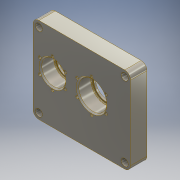
# Autodesk Inventor part: корпус01
Saved by Autodesk Inventor 2016 (Build 200138000, 138)
## iProperties
Created: 2021-04-22
Part Number: корпус01
Material: Типовые
Document SubType Name: Modeling
Designer: Лол
Density: 1 g/cm^3
Appearance: Титан — полированный
Author: Лол
Autodesk Inventor part; units mm, degrees
ref_plane "YZ Plane" through (0, 0, 0) normal (1, 0, 0) x (0, 1, 0)
ref_plane "XZ Plane" through (0, 0, 0) normal (0, 1, 0) x (-1, 0, 0)
ref_plane "XY Plane" through (0, 0, 0) normal (0, 0, 1) x (1, 0, 0)
sketch "Эскиз1" plane through (0, 0, 0) normal (0, 0, 1) x (1, 0, 0)
  line L0 (0, -65.4) -> (0, 10.9) projected
  line L1 (-170, 0) -> (180, 0) projected
  line L2 (-120, -12.5) -> (-120, -54.5)
  line L3 (-120, -54.5) -> (130, -54.5)
  line L4 (130, -54.5) -> (130, -12.5)
  line L5 (130, -12.5) -> (-120, -12.5)
  point P0 (0, 0)
  dimension "d0" = 12.5
  dimension "d1" = 250
  dimension "d2" = 42
  dimension "d3" = 120
  constraints: 8 end point, 3 perpendicular, 1 vertical
  measures "d0" distance between parallel lines of L5 L1
  measures "d1" distance of L2.end L3.end
  measures "d2" distance of L2.start L2.end
  measures "d3" distance between parallel lines of L2 L0
extrude "Выдавливание1" add sketch "Эскиз1" along normal blind 100 and the other way blind 120
sketch "Эскиз3" plane through (-120, -54.5, 100) normal (0, -1, 0) x (1, 0, 0)
  line L0 (120, -264) -> (120, 44) projected
  line L1 (-50, -100) -> (300, -100) projected
  circle A0 centre (150, -100) radius 36
  circle A1 centre (50, -100) radius 31
  point P0 (120, -100)
  dimension "d6" = 72
  dimension "d7" = 62
  dimension "d8" = 100
  dimension "d9" = 70
  constraints: 2 centre point, 2 point on line
  measures "d6" diameter of A0
  measures "d7" diameter of A1
  measures "d8" distance of A0.centre A1.centre
  measures "d9" distance from line of L0 A1.centre
extrude "Выдавливание2" cut sketch "Эскиз3" against normal blind 37
sketch "Эскиз4" plane through (-120, -54.5, 100) normal (0, -1, 0) x (1, 0, 0)
  line L0 (120, -264) -> (120, 44) projected
  line L1 (-50, -100) -> (300, -100) projected
  circle A0 centre (50, -100) radius 31 projected
  circle A1 centre (150, -100) radius 36 projected
  circle A2 centre (50, -100) radius 27
  circle A3 centre (150, -100) radius 31.5
  point P0 (120, -100)
  dimension "d12" = 63
  dimension "d13" = 54
  constraints: 2 centre point, 2 coincident
  measures "d12" diameter of A3
  measures "d13" diameter of A2
extrude "Выдавливание3" cut sketch "Эскиз4" against normal through all contours A3 L1 L0 | L0 L1 A3 | L1 A3 L0 | L0 A3 L1 | A2 L1 | L1 A2
sketch "Эскиз5" plane through (-120, -12.5, 100) normal (0, 1, 0) x (1, 0, 0)
  line L0 (120, 264) -> (120, -44) projected
  line L1 (-50, 100) -> (300, 100) projected
  circle A0 centre (150, 100) radius 31.5 projected
  circle A1 centre (50, 100) radius 27 projected
  arc A2 (86.0774, 126.8964) -> (86.0774, 73.1036) centre (50, 100) ccw
  arc A3 (108.2641, 72.4661) -> (108.2641, 127.5339) centre (150, 100) ccw
  arc A4 (86.0774, 126.8964) -> (108.2641, 127.5339) centre (96.9471, 135) ccw
  arc A5 (108.2641, 72.4661) -> (86.0774, 73.1036) centre (96.9471, 65) ccw
  line L2 (250, 220) -> (250, 0) projected
  line L3 (0, 220) -> (250, 220) projected
  line L4 (0, 0) -> (0, 220) projected
  line L5 (250, 0) -> (0, 0) projected
  line L6 (26, 214) -> (224, 214)
  line L7 (244, 194) -> (244, 26)
  line L8 (224, 6) -> (26, 6)
  line L9 (6, 26) -> (6, 194)
  arc A6 (244, 194) -> (224, 214) centre (224, 194) ccw
  arc A7 (26, 214) -> (6, 194) centre (26, 194) ccw
  arc A8 (6, 26) -> (26, 6) centre (26, 26) ccw
  arc A9 (224, 6) -> (244, 26) centre (224, 26) ccw
  point P0 (120, 100)
  dimension "d16" = 100
  dimension "d17" = 90
  dimension "d18" = 35
  dimension "d19" = 35
  dimension "d20" = 6
  dimension "d21" = 6
  dimension "d22" = 6
  dimension "d23" = 6
  dimension "d24" = 20
  constraints: 16 point on circle, 12 tangent, 8 centre point, 8 end point, 3 equal radius, 2 coincident, 2 parallel, 1 horizontal, 1 perpendicular
  measures "d16" diameter of A3
  measures "d17" diameter of A2
  measures "d18" distance from line of A4.centre L1
  measures "d19" distance from line of A5.centre L1
  measures "d20" distance between parallel lines of L7 L2
  measures "d21" distance between parallel lines of L3 L6
  measures "d22" distance between parallel lines of L4 L9
  measures "d23" distance between parallel lines of L5 L8
  measures "d24" radius of A6
extrude "Выдавливание4" cut sketch "Эскиз5" against normal blind 34 contours L6 A6 L7 L1 A3 L0 | L0 A3 A4 A2 L9 A7 L6 | L1 L7 A9 L8 L0 A3 | L0 L8 A8 L9 A2 A5 A3
fillet "Сопряжение1" radius 15 4 edges at (130, -33.5, -120) (130, -33.5, 100) (-120, -33.5, -120) (-120, -33.5, 100)
sketch "Эскиз7" plane through (-105, -12.5, 100) normal (0, 1, 0) x (1, 0, 0)
  arc A0 (220, 0) -> (235, 15) centre (220, 15) ccw projected
  arc A1 (-15, 15) -> (0, 0) centre (0, 15) ccw projected
  arc A2 (235, 205) -> (220, 220) centre (220, 205) ccw projected
  arc A3 (0, 220) -> (-15, 205) centre (0, 205) ccw projected
  circle A4 centre (220, 15) radius 15
  circle A5 centre (220, 205) radius 15
  circle A6 centre (0, 15) radius 15
  circle A7 centre (0, 205) radius 15
  point P0 (105, 100)
  constraints: 4 centre point, 4 coincident, 4 concentric
extrude "Выдавливание5" add sketch "Эскиз7" against normal blind 34
fillet "Сопряжение2" radius 10 2 edges at (-114, -29.5, 9.434) (-114, -29.5, -9.434)
fillet "Сопряжение3" radius 5 6 edges at (103, -29.5, -114) (124, -29.5, 73) (103, -29.5, 94) (-93, -29.5, 94) (-93, -29.5, -114) (-114, -29.5, -93)
sketch "Эскиз11" plane through (-105, -54.5, -120) normal (0, -1, 0) x (1, 0, 0)
  arc A0 (-9, 193) -> (14.6969, 208) centre (0, 205) ccw projected
  arc A1 (205.3031, 208) -> (223, 190.3031) centre (220, 205) ccw projected
  arc A2 (229, 27) -> (205.3031, 12) centre (220, 15) ccw projected
  arc A3 (14.6969, 12) -> (-3, 29.6969) centre (0, 15) ccw projected
  point P0 (105, 120)
  point P1 (-3, 190.3031)
  point P2 (223, 29.6969)
hole "Отверстие1" at (-105, -54.5, 85) at (115, -54.5, 85) at (115, -54.5, -105) at (-105, -54.5, -105) direction (0, 1, 0) diameter 10.2 depth 50 tip angle 118 counterbore diameter 18 counterbore depth 13.5
fillet "Сопряжение4" radius 15 2 edges at (-114, -29.5, 73) (124, -29.5, -93)
sketch "Эскиз12" plane through (-105, -12.5, 100) normal (0, 1, 0) x (1, 0, 0)
  circle A0 centre (220, 205) radius 5.1 projected
  circle A1 centre (0, 15) radius 5.1 projected
  circle A2 centre (225, 195) radius 3
  circle A3 centre (-5, 25) radius 3
  point P0 (105, 100)
  dimension "d54" = 6
  dimension "d55" = 10
  dimension "d57" = 5
  dimension "d58" = 230
  dimension "d59" = 170
  constraints: 2 centre point, 1 equal radius
  measures "d54" diameter of A3
  measures "d55" vertical distance of A2.centre A0.centre
  measures "d57" horizontal distance of A0.centre A2.centre
  measures "d58" horizontal distance of A3.centre A2.centre
  measures "d59" vertical distance of A3.centre A2.centre
hole "Отверстие2" at (120, -12.5, -95) at (-110, -12.5, 75) direction (0, -1, 0) diameter 6 depth 10 tip angle 118 countersink diameter 7.2 countersink angle 90
chamfer "Фаска2" distance 3.3 angle 45 1 edges at (-101, -54.5, 0)
chamfer "Фаска3" distance 3.3 angle 45 1 edges at (-6, -54.5, 0)
sketch "Эскиз13" plane through (-105, -54.5, -120) normal (0, -1, 0) x (1, 0, 0)
  circle A0 centre (35, 120) radius 31 projected
  circle A1 centre (35, 120) radius 37.5 construction
  line L0 (35, 120) -> (35, 157.5) construction
  circle A2 centre (35, 157.5) radius 1.5
  circle A3 centre (2.524, 138.75) radius 1.5
  circle A4 centre (2.524, 101.25) radius 1.5
  circle A5 centre (35, 82.5) radius 1.5
  circle A6 centre (67.476, 101.25) radius 1.5
  circle A7 centre (67.476, 138.75) radius 1.5
  point P0 (105, 120)
  dimension "d73" = 75
  dimension "d74" = 3
  dimension "d77" = 360
  constraints: 6 centre point, 2 coincident, 2 end point, 1 vertical, 1 vertical alignment, 15 other
  measures "d74" diameter of A2
hole "Отверстие3" at (-37.524, -54.5, 18.75) at (-70, -54.5, 37.5) at (-102.476, -54.5, 18.75) at (-102.476, -54.5, -18.75) at (-70, -54.5, -37.5) at (-37.524, -54.5, -18.75) direction (0, 1, 0) diameter 4.917 depth 15 tip angle 118 countersink diameter 7.2 countersink angle 90 thread size "M6x1" class "6H" standard "ISO Metric profile"
sketch "Эскиз14" plane through (0, 0, 0) normal (0, 0, 1) x (1, 0, 0)
  line L0 (-39, -51.2) -> (-39, -17.5) construction
  line L1 (-39, -17.5) -> (-101, -17.5) projected
  line L2 (-6, -51.2) -> (-6, -17.5) projected
  line L3 (66, -17.5) -> (-6, -17.5) projected
  line L4 (-39, -20.45) -> (-38.75, -20.2)
  line L5 (-38.75, -20.2) -> (-38.75, -17.2)
  line L6 (-43, -17.5) -> (-97, -17.5) projected
  line L7 (-38.75, -17.2) -> (-41.75, -17.2)
  line L8 (-41.75, -17.2) -> (-42.05, -17.5)
  line L9 (-42.05, -17.5) -> (-42.05, -20.45)
  line L10 (-42.05, -20.45) -> (-39, -20.45)
  line L11 (65.25, -21.2) -> (66.25, -20.2)
  line L12 (66.25, -20.2) -> (66.25, -17.2)
  line L13 (66.25, -17.2) -> (63.25, -17.2)
  line L14 (63.25, -17.2) -> (62.95, -17.5)
  line L15 (62.95, -17.5) -> (62.95, -21.2)
  line L16 (62.95, -21.2) -> (65.25, -21.2)
  line L17 (66, -51.2) -> (66, -17.5) projected
  line L18 (-70, -65.4037) -> (-70, 10.9006) projected
  line L19 (30, -65.4037) -> (30, 10.9006) projected
  point P0 (0, 0)
  dimension "d86" = 45
  dimension "d87" = 45
  dimension "d88" = 3
  dimension "d89" = 0.25
  dimension "d90" = 0.3
  dimension "d91" = 45
  dimension "d92" = 45
  dimension "d93" = 3
  dimension "d94" = 0.25
  dimension "d95" = 0.3
  dimension "d96" = 4
  constraints: 24 end point, 7 perpendicular, 3 point on line, 3 vertical
  measures "d86" angle of L0 L4
  measures "d87" angle of L1 L8
  measures "d88" distance from line of L4.end L7
  measures "d89" distance between parallel lines of L0 L5
  measures "d90" distance between parallel lines of L7 L1
  measures "d91" angle of L3 L14
  measures "d92" angle of L17 L11
  measures "d93" distance from line of L13 L11.end
  measures "d94" distance between parallel lines of L17 L12
  measures "d95" distance between parallel lines of L3 L13
  measures "d96" distance between parallel lines of L13 L16
revolve "Вращение1" cut sketch "Эскиз14" angle 360 about axis through (-70, -54.5, 0) along (0, 1, 0) contours L10 L9 L8 L7 L5 L4
revolve "Вращение2" cut sketch "Эскиз14" angle 360 about axis through (30, -54.5, 0) along (0, 1, 0) contours L17 L11 L16 L15 L3 | L3 L14 L13 L12 L11 L17
fillet "Сопряжение5" radius 1 2 edges at (-101.25, -17.2, 0) (-6.25, -17.2, 0)
fillet "Сопряжение6" radius 0.5 4 edges at (-101.25, -20.2, 0) (-98.25, -17.2, 0) (-3.25, -17.2, 0) (-6.25, -20.2, 0)
sketch "Эскиз15" plane through (-105, -54.5, -120) normal (0, -1, 0) x (1, 0, 0)
  circle A0 centre (135, 120) radius 36 projected
  circle A1 centre (135, 120) radius 36 projected
  line L0 (105, 264) -> (105, -44) projected
  line L1 (-65, 120) -> (285, 120) projected
  circle A2 centre (135, 120) radius 42.5 construction
  line L2 (135, 120) -> (135, 162.5) construction
  circle A3 centre (135, 162.5) radius 3
  point P0 (105, 120)
  dimension "d101" = 85
  dimension "d104" = 6
  dimension "d37" = 10.5
  constraints: 2 coincident, 2 end point, 1 centre point, 1 vertical, 1 vertical alignment, 2 other
  measures "d104" diameter of A3
hole "Отверстие4" at (30, -54.5, 42.5) direction (0, 1, 0) diameter 4.917 depth 15 tip angle 118 countersink diameter 7.2 countersink angle 90 thread size "M6x1" class "6H" standard "ISO Metric profile"
pattern_circular "Круговой массив1" count 6 over 360 about axis through (30, -54.5, 0) along (0, 1, 0) of "Отверстие4"
fillet "Сопряжение7" radius 5 24 edges at (-89.2771, -46.5, 92.1623) (-92.4864, -46.5, 76.729) (-110.619, -46.5, 65.093) (-114, -46.5, 49.419) (-108.3693, -46.5, 34.237) (-64.083, -46.5, 44.6093) (-22.6635, -46.5, 21.4477) (80, -46.5, 0) (-22.6635, -46.5, -21.4477) (-64.083, -46.5, -44.6093) (-108.3693, -46.5, -34.237) (-114, -46.5, -64.318) (-112.1623, -46.5, -89.2771) (-94.3934, -46.5, -94.3934) (-89.2771, -46.5, -112.1623) (5, -46.5, -114) (99.2771, -46.5, -112.1623) (102.4864, -46.5, -96.729) (120.619, -46.5, -85.093) (124, -46.5, -5.101) (122.1623, -46.5, 69.2771) (104.3934, -46.5, 74.3934) (99.2771, -46.5, 92.1623) (5, -46.5, 94)
